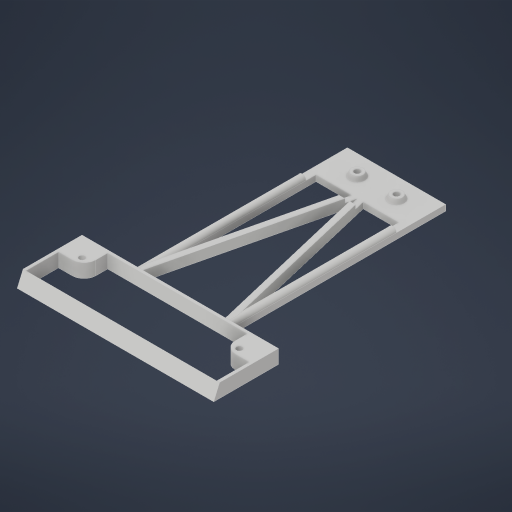
# Autodesk Inventor part: lf20cm
Saved by Autodesk Inventor 2023 (Build 270158000, 158)
## iProperties
Created: 2021-08-27
Part Number: lf20cm
Material: Ogólny
Document SubType Name: Modeling
Designer: Michał
Density: 1 g/cm^3
Appearance: Domyślna
Author: Michał
Autodesk Inventor part; units mm, degrees
ref_plane "YZ Plane" through (0, 0, 0) normal (1, 0, 0) x (0, 1, 0)
ref_plane "XZ Plane" through (0, 0, 0) normal (0, 1, 0) x (-1, 0, 0)
sketch "Szkic1" plane through (0, 0, 0) normal (0, 1, 0) x (-1, 0, 0)
  line L0 (0, 0) -> (-25, 0)
  line L1 (-25, 0) -> (-25, -110)
  line L2 (-25, -110) -> (0, -110)
  line L3 (0, -110) -> (0, 0)
  line L4 (-4, -2) -> (-25, -2)
  line L5 (-25, -2) -> (-25, -90)
  line L6 (-25, -90) -> (-4, -90)
  line L7 (-4, -90) -> (-4, -2)
  line L8 (-25, -90) -> (-4, -2)
  line L9 (-22, -90) -> (-4, -14.5714)
  line L10 (-4, -14.5714) -> (-4, -2)
  line L11 (-25, -90) -> (-22, -90)
  dimension "d0" = 25
  dimension "d1" = 110
  dimension "d2" = 4
  dimension "d3" = 20
  dimension "d4" = 2
  dimension "d7" = 3
  constraints: 24 end point, 5 parallel, 3 collinear, 2 horizontal, 2 perpendicular, 2 point on line
  measures "d0" distance of L2.end L1.end
  measures "d1" distance of L1.end L0.end
  measures "d2" distance between parallel lines of L3 L7
  measures "d3" distance between parallel lines of L2 L6
  measures "d4" distance between parallel lines of L0 L4
  measures "d7" distance of L9.start L5.end
extrude "Wyciągnięcie proste2" add sketch "Szkic1" along normal blind 5 contours L3 L2 L1 L6 L7 L4 L0 | L8 L7 L9 L6
sketch "Szkic2" plane through (25, 0, 0) normal (1, 0, 0) x (0, 0, -1)
  line L0 (0, 0) -> (-33, 0)
  line L1 (-33, 0) -> (-33, 7)
  line L2 (-33, 7) -> (0, 7)
  line L3 (0, 7) -> (0, 0)
  line L4 (-33, 0) -> (-30, 7)
  dimension "d10" = 33
  dimension "d11" = 7
  dimension "d12" = 30
  constraints: 10 end point, 2 parallel, 1 horizontal, 1 perpendicular, 1 point on line
  measures "d10" distance of L1.end L2.end
  measures "d11" distance of L0.end L1.end
  measures "d12" distance of L2.end L4.end
extrude "Wyciągnięcie proste3" add sketch "Szkic2" against normal blind 50 contours L0 L4 L2 L3
sketch "Szkic3" plane through (25, 7, 30) normal (0, 1, 0) x (1, 0, 0)
  line L0 (0, 0) -> (-50, 0) projected
  line L1 (0, 0) -> (-48.5, 0)
  line L2 (-48.5, 0) -> (-48.5, 28.5)
  line L3 (-48.5, 28.5) -> (0, 28.5)
  line L4 (-50, 0) -> (-50, 30) projected
  line L5 (-48.5, 28.5) -> (-41.5, 28.5)
  line L6 (-41.5, 28.5) -> (-41.5, 16.5)
  line L7 (-41.5, 16.5) -> (-48.5, 16.5)
  line L8 (-48.5, 16.5) -> (-48.5, 28.5)
  circle A0 centre (-41.5, 22.5) radius 6
  line L9 (-35.5, 22.5) -> (-41.5, 22.5)
  line L10 (-41.5, 22.5) -> (-41.5, 28.5)
  line L11 (-41.5, 28.5) -> (-35.5, 28.5)
  line L12 (-35.5, 28.5) -> (-35.5, 22.5)
  line L13 (0, 30) -> (-50, 30) projected
  line L14 (0, 30) -> (0, 0) projected
  line L15 (-19, 28.5) -> (-7, 28.5) construction
  line L16 (-22.5355, 28.5) -> (-19, 28.5)
  line L17 (-7, 28.5) -> (-5, 28.5)
  line L18 (-7, 0) -> (-5, 0)
  point P0 (-25, 30)
  dimension "d16" = 1.5
  dimension "d19" = 13
  dimension "d20" = 12
  dimension "d66" = 1.5
  constraints: 30 end point, 6 parallel, 4 horizontal, 3 perpendicular, 2 point on circle, 1 centre point, 1 midpoint, 1 point on line, 1 tangent
  measures "d16" distance between parallel lines of L4 L2
  measures "d19" distance between parallel lines of L8 L12
  measures "d20" distance between parallel lines of L3 L7
  measures "d66" distance between parallel lines of L13 L3
extrude "Wyciągnięcie proste4" cut sketch "Szkic3" against normal up to next contours L0 L2 L7 A0 L12 L3 L14
sketch "Szkic5" plane through (0, 5, 0) normal (0, 1, 0) x (1, 0, 0)
  line L0 (25, 90) -> (25, 110) projected
  line L1 (0, 110) -> (0, 0) projected
  line L2 (25, 110) -> (0, 110)
  line L3 (0, 110) -> (0, 85)
  line L4 (0, 85) -> (25, 85)
  line L5 (25, 85) -> (25, 110)
  circle A0 centre (15, 100) radius 3
  dimension "d30" = 25
  dimension "d31" = 6
  dimension "d32" = 10
  dimension "d33" = 10
  constraints: 8 end point, 2 parallel, 1 centre point, 1 horizontal, 1 perpendicular, 1 point on line
  measures "d30" distance between parallel lines of L2 L4
  measures "d31" diameter of A0
  measures "d32" distance from line of L0 A0.centre
  measures "d33" distance from line of L2 A0.centre
extrude "Wyciągnięcie proste6" cut sketch "Szkic5" against normal blind 2
chamfer "Faza2" distance 2 distance2 1 1 edges at (12, 3, -100) measured on face at (17.3983, 3.6667, -98.1978)
chamfer "Faza3" distance 2 angle 45 1 edges at (12.5, 5, 0)
sketch "Szkic6" plane through (15, 5, -100) normal (0, 1, 0) x (1, 0, 0)
  point P0 (-15, -100)
  point P1 (0, 0)
hole "Otwór1" at (15, 5, -100) direction (0, -1, 0) diameter 3 end through all
sketch "Szkic7" plane through (-25, 7, 30) normal (0, 1, 0) x (1, 0, 0)
  line L0 (14.5, 28.5) -> (14.5, 22.5) construction
  line L1 (14.5, 28.5) -> (14.5, 20) construction
  line L2 (14.5, 20) -> (1.5, 20) construction
  line L3 (1.5, 16.5) -> (1.5, 0) construction
  line L4 (1.5, 20) -> (1.5, 16.5) construction
  line L5 (1.5, 20) -> (10, 20) construction
  point P0 (25, 30)
  point P1 (14.5, 22.5)
  point P2 (12.5, 27.5)
  dimension "d49" = 8.5
  dimension "d50" = 8.5
  constraints: 8 end point, 1 coincident, 1 collinear, 1 perpendicular, 1 point on line, 1 vertical, 1 other
  measures "d49" distance of L1.start L1.end
  measures "d50" distance of L2.end L5.end
hole "Otwór2" at (-15, 7, 10) direction (0, -1, 0) diameter 3 end through all
ref_plane "Płaszczyzna konstrukcyjna1" through (25, 3, -48.75) normal (1, 0, 0) x (0, 0, 1)
mirror "Odbij1" about plane through (25, 3, -48.75) normal (1, 0, 0)
fillet "Fillet1" radius 2 4 edges at (4, 5, -49.7857) (0, 5, -43.4998) (46, 5, -49.7857) (50, 5, -43.4998)
